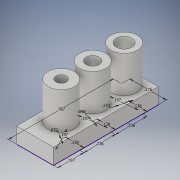
# Autodesk Inventor part: HoleSizeTest
Saved by Autodesk Inventor 2019 (Build 230136000, 136)
## iProperties
Created: 2019-05-04
Part Number: HoleSizeTest
Material: Generic
Document SubType Name: Modeling
Designer: Henry
Density: 1 g/cm^3
Appearance: Default
Author: Henry
Autodesk Inventor part; units mm, degrees
ref_plane "YZ Plane" through (0, 0, 0) normal (1, 0, 0) x (0, 1, 0)
ref_plane "XZ Plane" through (0, 0, 0) normal (0, 1, 0) x (-1, 0, 0)
ref_plane "XY Plane" through (0, 0, 0) normal (0, 0, 1) x (1, 0, 0)
sketch "Sketch1" plane through (0, 0, 0) normal (0, 1, 0) x (-1, 0, 0)
  line L0 (0, 0) -> (7, 0)
  line L1 (7, 0) -> (7, -20)
  line L2 (7, -20) -> (0, -20)
  line L3 (0, -20) -> (0, 0)
  line L4 (0, 0) -> (0, -5)
  line L5 (0, -5) -> (3.5, -5)
  circle A0 centre (3.5, -5) radius 2.5
  circle A1 centre (3.5, -5) radius 1
  line L6 (0, -5) -> (0, -11)
  line L7 (0, -11) -> (3.5, -11)
  circle A2 centre (3.5, -11) radius 2.5
  circle A3 centre (3.5, -11) radius 1.25
  line L8 (0, -11) -> (0, -17)
  line L9 (0, -17) -> (3.5, -17)
  circle A4 centre (3.5, -17) radius 2.5
  circle A5 centre (3.5, -17) radius 1.5
  dimension "d0" = 7
  dimension "d1" = 20
  dimension "d2" = 5
  dimension "d3" = 3.5
  dimension "d4" = 5
  dimension "d5" = 2
  dimension "d6" = 6
  dimension "d7" = 3.5
  dimension "d8" = 5
  dimension "d9" = 2.5
  dimension "d10" = 6
  dimension "d11" = 3.5
  dimension "d12" = 5
  dimension "d13" = 3
  constraints: 20 end point, 6 centre point, 6 coincident, 4 perpendicular, 3 point on line, 2 parallel, 1 horizontal
  measures "d0" distance of L1.end L2.end
  measures "d1" distance of L0.end L1.end
  measures "d2" distance of L0.start L4.end
  measures "d3" distance of L4.end L5.end
  measures "d4" diameter of A0
  measures "d5" diameter of A1
  measures "d6" distance of L4.end L6.end
  measures "d7" distance of L6.end L7.end
  measures "d8" diameter of A2
  measures "d9" diameter of A3
  measures "d10" distance of L6.end L8.end
  measures "d11" distance of L8.end L9.end
  measures "d12" diameter of A4
  measures "d13" diameter of A5
extrude "Extrusion1" add sketch "Sketch1" along normal blind 3 contours L0 L1 L2 L3
extrude "Extrusion2" add sketch "Sketch1" along normal blind 3 contours A1 | A3 | A5
extrude "Extrusion3" add sketch "Sketch1" along normal blind 10 contours A0 | A2 | A4
body "Solid1"
